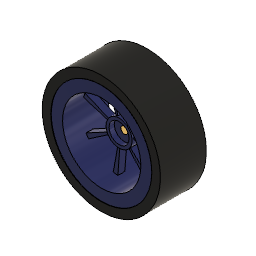
Wheel (Autodesk Fusion 360 design; units mm, degrees)
part number: 2026-02-05-15-46-21-307
Autodesk Fusion 360 part; units mm, degrees
sketch "Sketch1" plane through (0, 0, 0) normal (0, 1, 0) x (1, 0, 0)
  circle A0 centre (0, 0) radius 34
  circle A1 centre (0, 0) radius 29
  circle A2 centre (0, 0) radius 22.5
  circle A3 centre (0, 0) radius 5.75
  circle A4 centre (0, 0) radius 2
  circle A5 centre (0, 0) radius 7.5
  line L0 (4.6641, -5.8734) -> (13.4973, -18.002)
  line L1 (3.7575, -6.4909) -> (11.2724, -19.4726)
  line L2 (7.4175, -1.1093) -> (22.2525, -3.3279)
  line L3 (7.5, -0.0155) -> (22.49, -0.6714)
  line L4 (5.492, 5.1076) -> (16.4761, 15.3228)
  line L5 (4.6882, 5.8541) -> (14.5472, 17.1648)
  line L6 (-0.5691, 7.4784) -> (-1.7072, 22.4351)
  line L7 (-1.6538, 7.3154) -> (-4.3499, 22.0755)
  line L8 (-6.2016, 4.2178) -> (-18.6049, 12.6533)
  line L9 (-6.7505, 3.268) -> (-19.9715, 10.363)
  line L10 (-7.1643, -2.2189) -> (-21.4928, -6.6567)
  line L11 (-6.764, -3.2402) -> (-20.5541, -9.1531)
  line L12 (-2.732, -6.9847) -> (-8.1961, -20.9541)
  line L13 (-1.684, -7.3085) -> (-5.6591, -21.7767)
  dimension "d1" = 68
  dimension "d2" = 58
  dimension "d3" = 45
  dimension "d4" = 11.5
  dimension "d5" = 4
  dimension "d6" = 15
  dimension "d8" = 6
  dimension "d10" = 360
  constraint coincident A0.centre A1.centre
  constraint concentric A0 A3
  constraint concentric A2 A5
  constraint coincident A5 L0.start
  constraint coincident A2 L0.end
  constraint coincident A5 L1.start
  constraint coincident A0.centre L1
  constraint coincident A2 L1.end
  measures "d1" diameter of A0
  measures "d2" diameter of A1
  measures "d3" diameter of A2
  measures "d4" diameter of A3
  measures "d5" diameter of A4
  measures "d6" diameter of A5
  measures "d8" angle of L0 L1
extrude "Extrude1" add sketch "Sketch1" along normal blind 17.5 contours A3 makes body 1
extrude "Extrude2" add sketch "Sketch1" along normal mid plane 6 contours A5 bodies 1
extrude "Extrude3" add sketch "Sketch1" along normal mid plane 4 contours A2 A5 L4 L5 | A2 A5 L2 L3 | A2 A5 L6 L7 | A2 A5 L0 L1 | A2 A5 L8 L9 | A2 A5 L12 L13 | A2 A5 L10 L11 bodies 1
extrude "Extrude4" add sketch "Sketch1" along normal mid plane 26.5 separate body contours A0 makes body 2
extrude "Extrude5" add sketch "Sketch1" along normal mid plane 26 contours A1 bodies 1 2
equation "d11 = 3 mm + 14.5 mm"
